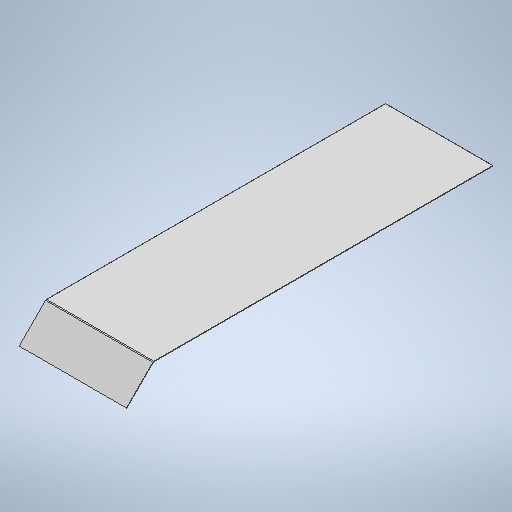
# Autodesk Inventor part: BSH 013 floor
Saved by Autodesk Inventor 2025 (Build 290162010, 162A)
## iProperties
Created: 2024-07-23
Part Number: BSH 013 floor
Material: 09g2s
Document SubType Name: Sheet Metal
Designer: admin
Mass: 81987.7 g
Surface Area: 69857.9 cm^2
Volume: 10444.3 cm^3
Density: 7.85 g/cm^3
Flat Pattern Width: 60 cm
Flat Pattern Length: 211.034 cm
Flat Pattern Area: 12662 cm^2
Sheet Metal Rule: AISI304 3mm Die 32
Sheet Metal Width: 600,000 mm
Sheet Metal Length: 2110,336 mm
Sheet Metal Area: 1266201,780 mm^2
Appearance: Default
Stock Number: БШК 013 пол
Author: admin
Autodesk Inventor part; units mm, degrees
ref_plane "YZ Plane" through (0, 0, 0) normal (1, 0, 0) x (0, 1, 0)
ref_plane "XZ Plane" through (0, 0, 0) normal (0, 1, 0) x (-1, 0, 0)
ref_plane "XY Plane" through (0, 0, 0) normal (0, 0, 1) x (1, 0, 0)
sketch "Sketch1" plane through (0, 0, 0) normal (0, 0, 1) x (1, 0, 0)
  line L0 (-300, -950) -> (300, -950)
  line L1 (300, -950) -> (300, 950)
  line L2 (300, 950) -> (-300, 950)
  line L3 (-300, 950) -> (-300, -950)
  line L4 (-300, -950) -> (300, 950) construction
  line L5 (300, -950) -> (-300, 950) construction
  point P0 (0, 0)
  dimension "d0" = 600
  dimension "d1" = 1900
  measures "d0" distance of L2.end L1.end
  measures "d1" distance of L1.end L0.end
extrude "Plate1" add sketch "Sketch1" along normal blind 3
sketch "Sketch3" plane through (-300, -947.8787, 0.8787) normal (0, -0.7071068, 0.7071068) x (1, 0, 0)
  line L0 (600, 0) -> (0, 0)
  line L1 (0, 0) -> (0, -212)
  line L2 (0, -212) -> (600, -212)
  line L3 (600, -212) -> (600, 0)
  constraints: 6 end point, 1 horizontal, 1 perpendicular, 1 vertical
edge flange "Flange2" height 212 angle 45 thickness 3 bend radius 5 thickness toward (0, -0.7071068, 0.7071068) relief round relief width 3 relief depth 1.5 edges at (0, -950, 0) wall of the first edge with corners at (300, -947.8787, 0.8787) (-300, -947.8787, 0.8787) (-300, -1097.7853, -149.028) (300, -1097.7853, -149.028)
bend "Bend2"
corner "Corner2"
sketch "Sketch5" plane through (300, -1097.7853, -149.028) normal (0, 0.7071068, -0.7071068) x (-1, 0, 0)
  line L0 (575, 36.661) -> (575, 25) construction
  line L1 (575, 25) -> (375, 25) construction
  line L2 (375, 25) -> (375, 36.661) construction
  line L3 (375, 36.661) -> (575, 36.661) construction
  line L4 (0, 0) -> (600, 0) projected
  line L5 (600, 208.6863) -> (600, 0) projected
  point P0 (300, 881.6301)
  point P1 (575, 30.8305)
  dimension "d23" = 200
  dimension "d24" = 11.661
  dimension "d25" = 25
  dimension "d26" = 25
  constraints: 1 midpoint, 2 other
  measures "d23" distance of L0.end L1.end
  measures "d24" distance between parallel lines of L1 L3
  measures "d25" distance between parallel lines of L4 L1
  measures "d26" distance between parallel lines of L5 L0
mark "Mark1"
equation "\"d2\" = Thickness"
equation "\"d13\" = BendReliefWidth"
equation "\"d14\" = BendReliefDepth"
equation "\"d15\" = MinimumRemnant"
equation "\"d16\" = TransitionRadius"
equation "\"d19\" = BendRadius"
equation "\"d20\" = CornerReliefSize"
equation "\"d21\" = GapSize"
equation "\"d22\" = JacobiRadiusSize"
equation "\"BendReliefWidth\" = Thickness"
equation "\"BendReliefDepth\" = 0.5 * Thickness"
equation "\"CornerReliefSize\" = 4 * Thickness"
equation "\"MinimumRemnant\" = 2 * Thickness"
equation "\"TransitionRadius\" = BendRadius"
equation "\"JacobiRadiusSize\" = BendRadius"
equation "\"GapSize\" = Thickness"
equation "\"Thickness\" = 3"
equation "\"BendRadius\" = 5"
body "Solid1"
